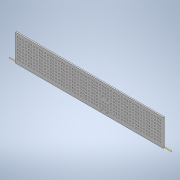
# Autodesk Inventor part: top_plate
Saved by Autodesk Inventor 2022 (Build 260153000, 153)
## iProperties
Created: 2021-07-14
Part Number: top_plate
Material: Generic
Document SubType Name: Modeling
Designer: gfellows
Density: 1 g/cm^3
Appearance: Default
Author: gfellows
Autodesk Inventor part; units mm, degrees
ref_plane "YZ Plane" through (0, 0, 0) normal (1, 0, 0) x (0, 1, 0)
ref_plane "XZ Plane" through (0, 0, 0) normal (0, 1, 0) x (-1, 0, 0)
ref_plane "XY Plane" through (0, 0, 0) normal (0, 0, 1) x (1, 0, 0)
ref_plane "Work Plane1" through (-371.7905, 0, 55) normal (0, 0, 1) x (1, 0, 0)
sketch "Sketch1" plane through (-371.7905, 0, 55) normal (0, 0, 1) x (1, 0, 0)
  line L0 (0, 0) -> (430.2, 0)
  line L1 (430.2, 0) -> (430.2, 78.35)
  line L2 (430.2, 78.35) -> (0, 78.35)
  line L3 (0, 78.35) -> (0, 0)
  circle A0 centre (265.5182, 6.225) radius 1.3525 projected
  line L4 (232.7522, 3.429) -> (232.7522, 41.021) projected
  line L5 (271.9952, 3.429) -> (232.7522, 3.429) projected
  line L6 (271.9952, 41.021) -> (271.9952, 3.429) projected
  line L7 (232.7522, 41.021) -> (271.9952, 41.021) projected
  circle A1 centre (265.5182, 6.225) radius 1.3525 projected
  circle A2 centre (249.5182, 6.225) radius 1.3525 projected
  circle A3 centre (265.5182, 38.225) radius 1.3525 projected
  circle A4 centre (249.5182, 38.225) radius 1.3525 projected
  circle A5 centre (5.8257, 12.35) radius 1.65
  line L8 (0, 75.175) -> (0, 78.35) projected
  line L9 (0, 0) -> (430.2, 0) projected
  circle A6 centre (5.8257, 20.35) radius 1.65
  circle A7 centre (5.8257, 28.35) radius 1.65
  circle A8 centre (5.8257, 36.35) radius 1.65
  circle A9 centre (5.8257, 44.35) radius 1.65
  circle A10 centre (5.8257, 52.35) radius 1.65
  circle A11 centre (5.8257, 60.35) radius 1.65
  circle A12 centre (5.8257, 68.35) radius 1.65
  circle A13 centre (13.8257, 12.35) radius 1.65
  circle A14 centre (13.8257, 20.35) radius 1.65
  circle A15 centre (13.8257, 28.35) radius 1.65
  circle A16 centre (13.8257, 36.35) radius 1.65
  circle A17 centre (13.8257, 44.35) radius 1.65
  circle A18 centre (13.8257, 52.35) radius 1.65
  circle A19 centre (13.8257, 60.35) radius 1.65
  circle A20 centre (13.8257, 68.35) radius 1.65
  circle A21 centre (21.8257, 12.35) radius 1.65
  circle A22 centre (21.8257, 20.35) radius 1.65
  circle A23 centre (21.8257, 28.35) radius 1.65
  circle A24 centre (21.8257, 36.35) radius 1.65
  circle A25 centre (21.8257, 44.35) radius 1.65
  circle A26 centre (21.8257, 52.35) radius 1.65
  circle A27 centre (21.8257, 60.35) radius 1.65
  circle A28 centre (21.8257, 68.35) radius 1.65
  circle A29 centre (29.8257, 12.35) radius 1.65
  circle A30 centre (29.8257, 20.35) radius 1.65
  circle A31 centre (29.8257, 28.35) radius 1.65
  circle A32 centre (29.8257, 36.35) radius 1.65
  circle A33 centre (29.8257, 44.35) radius 1.65
  circle A34 centre (29.8257, 52.35) radius 1.65
  circle A35 centre (29.8257, 60.35) radius 1.65
  circle A36 centre (29.8257, 68.35) radius 1.65
  circle A37 centre (37.8257, 12.35) radius 1.65
  circle A38 centre (37.8257, 20.35) radius 1.65
  circle A39 centre (37.8257, 28.35) radius 1.65
  circle A40 centre (37.8257, 36.35) radius 1.65
  circle A41 centre (37.8257, 44.35) radius 1.65
  circle A42 centre (37.8257, 52.35) radius 1.65
  circle A43 centre (37.8257, 60.35) radius 1.65
  circle A44 centre (37.8257, 68.35) radius 1.65
  circle A45 centre (45.8257, 12.35) radius 1.65
  circle A46 centre (45.8257, 20.35) radius 1.65
  circle A47 centre (45.8257, 28.35) radius 1.65
  circle A48 centre (45.8257, 36.35) radius 1.65
  circle A49 centre (45.8257, 44.35) radius 1.65
  circle A50 centre (45.8257, 52.35) radius 1.65
  circle A51 centre (45.8257, 60.35) radius 1.65
  circle A52 centre (45.8257, 68.35) radius 1.65
  circle A53 centre (53.8257, 12.35) radius 1.65
  circle A54 centre (53.8257, 20.35) radius 1.65
  circle A55 centre (53.8257, 28.35) radius 1.65
  circle A56 centre (53.8257, 36.35) radius 1.65
  circle A57 centre (53.8257, 44.35) radius 1.65
  circle A58 centre (53.8257, 52.35) radius 1.65
  circle A59 centre (53.8257, 60.35) radius 1.65
  circle A60 centre (53.8257, 68.35) radius 1.65
  circle A61 centre (61.8257, 12.35) radius 1.65
  circle A62 centre (61.8257, 20.35) radius 1.65
  circle A63 centre (61.8257, 28.35) radius 1.65
  circle A64 centre (61.8257, 36.35) radius 1.65
  circle A65 centre (61.8257, 44.35) radius 1.65
  circle A66 centre (61.8257, 52.35) radius 1.65
  circle A67 centre (61.8257, 60.35) radius 1.65
  circle A68 centre (61.8257, 68.35) radius 1.65
  circle A69 centre (69.8257, 12.35) radius 1.65
  circle A70 centre (69.8257, 20.35) radius 1.65
  circle A71 centre (69.8257, 28.35) radius 1.65
  circle A72 centre (69.8257, 36.35) radius 1.65
  circle A73 centre (69.8257, 44.35) radius 1.65
  circle A74 centre (69.8257, 52.35) radius 1.65
  circle A75 centre (69.8257, 60.35) radius 1.65
  circle A76 centre (69.8257, 68.35) radius 1.65
  circle A77 centre (77.8257, 12.35) radius 1.65
  circle A78 centre (77.8257, 20.35) radius 1.65
  circle A79 centre (77.8257, 28.35) radius 1.65
  circle A80 centre (77.8257, 36.35) radius 1.65
  circle A81 centre (77.8257, 44.35) radius 1.65
  circle A82 centre (77.8257, 52.35) radius 1.65
  circle A83 centre (77.8257, 60.35) radius 1.65
  circle A84 centre (77.8257, 68.35) radius 1.65
  circle A85 centre (85.8257, 12.35) radius 1.65
  circle A86 centre (85.8257, 20.35) radius 1.65
  circle A87 centre (85.8257, 28.35) radius 1.65
  circle A88 centre (85.8257, 36.35) radius 1.65
  circle A89 centre (85.8257, 44.35) radius 1.65
  circle A90 centre (85.8257, 52.35) radius 1.65
  circle A91 centre (85.8257, 60.35) radius 1.65
  circle A92 centre (85.8257, 68.35) radius 1.65
  circle A93 centre (93.8257, 12.35) radius 1.65
  circle A94 centre (93.8257, 20.35) radius 1.65
  circle A95 centre (93.8257, 28.35) radius 1.65
  circle A96 centre (93.8257, 36.35) radius 1.65
  circle A97 centre (93.8257, 44.35) radius 1.65
  circle A98 centre (93.8257, 52.35) radius 1.65
  circle A99 centre (93.8257, 60.35) radius 1.65
  circle A100 centre (93.8257, 68.35) radius 1.65
  circle A101 centre (101.8257, 12.35) radius 1.65
  circle A102 centre (101.8257, 20.35) radius 1.65
  circle A103 centre (101.8257, 28.35) radius 1.65
  circle A104 centre (101.8257, 36.35) radius 1.65
  circle A105 centre (101.8257, 44.35) radius 1.65
  circle A106 centre (101.8257, 52.35) radius 1.65
  circle A107 centre (101.8257, 60.35) radius 1.65
  circle A108 centre (101.8257, 68.35) radius 1.65
  circle A109 centre (109.8257, 12.35) radius 1.65
  circle A110 centre (109.8257, 20.35) radius 1.65
  circle A111 centre (109.8257, 28.35) radius 1.65
  circle A112 centre (109.8257, 36.35) radius 1.65
  circle A113 centre (109.8257, 44.35) radius 1.65
  circle A114 centre (109.8257, 52.35) radius 1.65
  circle A115 centre (109.8257, 60.35) radius 1.65
  circle A116 centre (109.8257, 68.35) radius 1.65
  circle A117 centre (117.8257, 12.35) radius 1.65
  circle A118 centre (117.8257, 20.35) radius 1.65
  circle A119 centre (117.8257, 28.35) radius 1.65
  circle A120 centre (117.8257, 36.35) radius 1.65
  circle A121 centre (117.8257, 44.35) radius 1.65
  circle A122 centre (117.8257, 52.35) radius 1.65
  circle A123 centre (117.8257, 60.35) radius 1.65
  circle A124 centre (117.8257, 68.35) radius 1.65
  circle A125 centre (125.8257, 12.35) radius 1.65
  circle A126 centre (125.8257, 20.35) radius 1.65
  circle A127 centre (125.8257, 28.35) radius 1.65
  circle A128 centre (125.8257, 36.35) radius 1.65
  circle A129 centre (125.8257, 44.35) radius 1.65
  circle A130 centre (125.8257, 52.35) radius 1.65
  circle A131 centre (125.8257, 60.35) radius 1.65
  circle A132 centre (125.8257, 68.35) radius 1.65
  circle A133 centre (133.8257, 12.35) radius 1.65
  circle A134 centre (133.8257, 20.35) radius 1.65
  circle A135 centre (133.8257, 28.35) radius 1.65
  circle A136 centre (133.8257, 36.35) radius 1.65
  circle A137 centre (133.8257, 44.35) radius 1.65
  circle A138 centre (133.8257, 52.35) radius 1.65
  circle A139 centre (133.8257, 60.35) radius 1.65
  circle A140 centre (133.8257, 68.35) radius 1.65
  circle A141 centre (141.8257, 12.35) radius 1.65
  circle A142 centre (141.8257, 20.35) radius 1.65
  circle A143 centre (141.8257, 28.35) radius 1.65
  circle A144 centre (141.8257, 36.35) radius 1.65
  circle A145 centre (141.8257, 44.35) radius 1.65
  circle A146 centre (141.8257, 52.35) radius 1.65
  circle A147 centre (141.8257, 60.35) radius 1.65
  circle A148 centre (141.8257, 68.35) radius 1.65
  circle A149 centre (149.8257, 12.35) radius 1.65
  circle A150 centre (149.8257, 20.35) radius 1.65
  circle A151 centre (149.8257, 28.35) radius 1.65
  circle A152 centre (149.8257, 36.35) radius 1.65
  circle A153 centre (149.8257, 44.35) radius 1.65
  circle A154 centre (149.8257, 52.35) radius 1.65
  circle A155 centre (149.8257, 60.35) radius 1.65
  circle A156 centre (149.8257, 68.35) radius 1.65
  circle A157 centre (157.8257, 12.35) radius 1.65
  circle A158 centre (157.8257, 20.35) radius 1.65
  circle A159 centre (157.8257, 28.35) radius 1.65
  circle A160 centre (157.8257, 36.35) radius 1.65
  circle A161 centre (157.8257, 44.35) radius 1.65
  circle A162 centre (157.8257, 52.35) radius 1.65
  circle A163 centre (157.8257, 60.35) radius 1.65
  circle A164 centre (157.8257, 68.35) radius 1.65
  circle A165 centre (165.8257, 12.35) radius 1.65
  circle A166 centre (165.8257, 20.35) radius 1.65
  circle A167 centre (165.8257, 28.35) radius 1.65
  circle A168 centre (165.8257, 36.35) radius 1.65
  circle A169 centre (165.8257, 44.35) radius 1.65
  circle A170 centre (165.8257, 52.35) radius 1.65
  circle A171 centre (165.8257, 60.35) radius 1.65
  circle A172 centre (165.8257, 68.35) radius 1.65
  circle A173 centre (173.8257, 12.35) radius 1.65
  circle A174 centre (173.8257, 20.35) radius 1.65
  circle A175 centre (173.8257, 28.35) radius 1.65
  circle A176 centre (173.8257, 36.35) radius 1.65
  circle A177 centre (173.8257, 44.35) radius 1.65
  circle A178 centre (173.8257, 52.35) radius 1.65
  circle A179 centre (173.8257, 60.35) radius 1.65
  circle A180 centre (173.8257, 68.35) radius 1.65
  circle A181 centre (181.8257, 12.35) radius 1.65
  circle A182 centre (181.8257, 20.35) radius 1.65
  circle A183 centre (181.8257, 28.35) radius 1.65
  circle A184 centre (181.8257, 36.35) radius 1.65
  circle A185 centre (181.8257, 44.35) radius 1.65
  circle A186 centre (181.8257, 52.35) radius 1.65
  circle A187 centre (181.8257, 60.35) radius 1.65
  circle A188 centre (181.8257, 68.35) radius 1.65
  circle A189 centre (189.8257, 12.35) radius 1.65
  circle A190 centre (189.8257, 20.35) radius 1.65
  circle A191 centre (189.8257, 28.35) radius 1.65
  circle A192 centre (189.8257, 36.35) radius 1.65
  circle A193 centre (189.8257, 44.35) radius 1.65
  circle A194 centre (189.8257, 52.35) radius 1.65
  circle A195 centre (189.8257, 60.35) radius 1.65
  circle A196 centre (189.8257, 68.35) radius 1.65
  circle A197 centre (197.8257, 12.35) radius 1.65
  circle A198 centre (197.8257, 20.35) radius 1.65
  circle A199 centre (197.8257, 28.35) radius 1.65
  circle A200 centre (197.8257, 36.35) radius 1.65
  circle A201 centre (197.8257, 44.35) radius 1.65
  circle A202 centre (197.8257, 52.35) radius 1.65
  circle A203 centre (197.8257, 60.35) radius 1.65
  circle A204 centre (197.8257, 68.35) radius 1.65
  circle A205 centre (205.8257, 12.35) radius 1.65
  circle A206 centre (205.8257, 20.35) radius 1.65
  circle A207 centre (205.8257, 28.35) radius 1.65
  circle A208 centre (205.8257, 36.35) radius 1.65
  circle A209 centre (205.8257, 44.35) radius 1.65
  circle A210 centre (205.8257, 52.35) radius 1.65
  circle A211 centre (205.8257, 60.35) radius 1.65
  circle A212 centre (205.8257, 68.35) radius 1.65
  circle A213 centre (213.8257, 12.35) radius 1.65
  circle A214 centre (213.8257, 20.35) radius 1.65
  circle A215 centre (213.8257, 28.35) radius 1.65
  circle A216 centre (213.8257, 36.35) radius 1.65
  circle A217 centre (213.8257, 44.35) radius 1.65
  circle A218 centre (213.8257, 52.35) radius 1.65
  circle A219 centre (213.8257, 60.35) radius 1.65
  circle A220 centre (213.8257, 68.35) radius 1.65
  circle A221 centre (221.8257, 12.35) radius 1.65
  circle A222 centre (221.8257, 20.35) radius 1.65
  circle A223 centre (221.8257, 28.35) radius 1.65
  circle A224 centre (221.8257, 36.35) radius 1.65
  circle A225 centre (221.8257, 44.35) radius 1.65
  circle A226 centre (221.8257, 52.35) radius 1.65
  circle A227 centre (221.8257, 60.35) radius 1.65
  circle A228 centre (221.8257, 68.35) radius 1.65
  circle A229 centre (229.8257, 12.35) radius 1.65
  circle A230 centre (229.8257, 20.35) radius 1.65
  circle A231 centre (229.8257, 28.35) radius 1.65
  circle A232 centre (229.8257, 36.35) radius 1.65
  circle A233 centre (229.8257, 44.35) radius 1.65
  circle A234 centre (229.8257, 52.35) radius 1.65
  circle A235 centre (229.8257, 60.35) radius 1.65
  circle A236 centre (229.8257, 68.35) radius 1.65
  circle A237 centre (237.8257, 12.35) radius 1.65
  circle A238 centre (237.8257, 20.35) radius 1.65
  circle A239 centre (237.8257, 28.35) radius 1.65
  circle A240 centre (237.8257, 36.35) radius 1.65
  circle A241 centre (237.8257, 44.35) radius 1.65
  circle A242 centre (237.8257, 52.35) radius 1.65
  circle A243 centre (237.8257, 60.35) radius 1.65
  circle A244 centre (237.8257, 68.35) radius 1.65
  circle A245 centre (245.8257, 12.35) radius 1.65
  circle A246 centre (245.8257, 20.35) radius 1.65
  circle A247 centre (245.8257, 28.35) radius 1.65
  circle A248 centre (245.8257, 36.35) radius 1.65
  circle A249 centre (245.8257, 44.35) radius 1.65
  circle A250 centre (245.8257, 52.35) radius 1.65
  circle A251 centre (245.8257, 60.35) radius 1.65
  circle A252 centre (245.8257, 68.35) radius 1.65
  circle A253 centre (253.8257, 12.35) radius 1.65
  circle A254 centre (253.8257, 20.35) radius 1.65
  circle A255 centre (253.8257, 28.35) radius 1.65
  circle A256 centre (253.8257, 36.35) radius 1.65
  circle A257 centre (253.8257, 44.35) radius 1.65
  circle A258 centre (253.8257, 52.35) radius 1.65
  circle A259 centre (253.8257, 60.35) radius 1.65
  circle A260 centre (253.8257, 68.35) radius 1.65
  circle A261 centre (261.8257, 12.35) radius 1.65
  circle A262 centre (261.8257, 20.35) radius 1.65
  circle A263 centre (261.8257, 28.35) radius 1.65
  circle A264 centre (261.8257, 36.35) radius 1.65
  circle A265 centre (261.8257, 44.35) radius 1.65
  circle A266 centre (261.8257, 52.35) radius 1.65
  circle A267 centre (261.8257, 60.35) radius 1.65
  circle A268 centre (261.8257, 68.35) radius 1.65
  circle A269 centre (269.8257, 12.35) radius 1.65
  circle A270 centre (269.8257, 20.35) radius 1.65
  circle A271 centre (269.8257, 28.35) radius 1.65
  circle A272 centre (269.8257, 36.35) radius 1.65
  circle A273 centre (269.8257, 44.35) radius 1.65
  circle A274 centre (269.8257, 52.35) radius 1.65
  circle A275 centre (269.8257, 60.35) radius 1.65
  circle A276 centre (269.8257, 68.35) radius 1.65
  circle A277 centre (277.8257, 12.35) radius 1.65
  circle A278 centre (277.8257, 20.35) radius 1.65
  circle A279 centre (277.8257, 28.35) radius 1.65
  circle A280 centre (277.8257, 36.35) radius 1.65
  circle A281 centre (277.8257, 44.35) radius 1.65
  circle A282 centre (277.8257, 52.35) radius 1.65
  circle A283 centre (277.8257, 60.35) radius 1.65
  circle A284 centre (277.8257, 68.35) radius 1.65
  circle A285 centre (285.8257, 12.35) radius 1.65
  circle A286 centre (285.8257, 20.35) radius 1.65
  circle A287 centre (285.8257, 28.35) radius 1.65
  circle A288 centre (285.8257, 36.35) radius 1.65
  circle A289 centre (285.8257, 44.35) radius 1.65
  circle A290 centre (285.8257, 52.35) radius 1.65
  circle A291 centre (285.8257, 60.35) radius 1.65
  circle A292 centre (285.8257, 68.35) radius 1.65
  circle A293 centre (293.8257, 12.35) radius 1.65
  circle A294 centre (293.8257, 20.35) radius 1.65
  circle A295 centre (293.8257, 28.35) radius 1.65
  circle A296 centre (293.8257, 36.35) radius 1.65
  circle A297 centre (293.8257, 44.35) radius 1.65
  circle A298 centre (293.8257, 52.35) radius 1.65
  circle A299 centre (293.8257, 60.35) radius 1.65
  circle A300 centre (293.8257, 68.35) radius 1.65
  circle A301 centre (301.8257, 12.35) radius 1.65
  circle A302 centre (301.8257, 20.35) radius 1.65
  circle A303 centre (301.8257, 28.35) radius 1.65
  circle A304 centre (301.8257, 36.35) radius 1.65
  circle A305 centre (301.8257, 44.35) radius 1.65
  circle A306 centre (301.8257, 52.35) radius 1.65
  circle A307 centre (301.8257, 60.35) radius 1.65
  circle A308 centre (301.8257, 68.35) radius 1.65
  circle A309 centre (309.8257, 12.35) radius 1.65
  circle A310 centre (309.8257, 20.35) radius 1.65
  circle A311 centre (309.8257, 28.35) radius 1.65
  circle A312 centre (309.8257, 36.35) radius 1.65
  circle A313 centre (309.8257, 44.35) radius 1.65
  circle A314 centre (309.8257, 52.35) radius 1.65
  circle A315 centre (309.8257, 60.35) radius 1.65
  circle A316 centre (309.8257, 68.35) radius 1.65
  circle A317 centre (317.8257, 12.35) radius 1.65
  circle A318 centre (317.8257, 20.35) radius 1.65
  circle A319 centre (317.8257, 28.35) radius 1.65
  circle A320 centre (317.8257, 36.35) radius 1.65
  circle A321 centre (317.8257, 44.35) radius 1.65
  circle A322 centre (317.8257, 52.35) radius 1.65
  circle A323 centre (317.8257, 60.35) radius 1.65
  circle A324 centre (317.8257, 68.35) radius 1.65
  circle A325 centre (325.8257, 12.35) radius 1.65
  circle A326 centre (325.8257, 20.35) radius 1.65
  circle A327 centre (325.8257, 28.35) radius 1.65
  circle A328 centre (325.8257, 36.35) radius 1.65
  circle A329 centre (325.8257, 44.35) radius 1.65
  circle A330 centre (325.8257, 52.35) radius 1.65
  circle A331 centre (325.8257, 60.35) radius 1.65
  circle A332 centre (325.8257, 68.35) radius 1.65
  circle A333 centre (333.8257, 12.35) radius 1.65
  circle A334 centre (333.8257, 20.35) radius 1.65
  circle A335 centre (333.8257, 28.35) radius 1.65
  circle A336 centre (333.8257, 36.35) radius 1.65
  circle A337 centre (333.8257, 44.35) radius 1.65
  circle A338 centre (333.8257, 52.35) radius 1.65
  circle A339 centre (333.8257, 60.35) radius 1.65
  circle A340 centre (333.8257, 68.35) radius 1.65
  circle A341 centre (341.8257, 12.35) radius 1.65
  circle A342 centre (341.8257, 20.35) radius 1.65
  circle A343 centre (341.8257, 28.35) radius 1.65
  circle A344 centre (341.8257, 36.35) radius 1.65
  circle A345 centre (341.8257, 44.35) radius 1.65
  circle A346 centre (341.8257, 52.35) radius 1.65
  circle A347 centre (341.8257, 60.35) radius 1.65
  circle A348 centre (341.8257, 68.35) radius 1.65
  circle A349 centre (349.8257, 12.35) radius 1.65
  circle A350 centre (349.8257, 20.35) radius 1.65
  circle A351 centre (349.8257, 28.35) radius 1.65
  circle A352 centre (349.8257, 36.35) radius 1.65
  circle A353 centre (349.8257, 44.35) radius 1.65
  circle A354 centre (349.8257, 52.35) radius 1.65
  circle A355 centre (349.8257, 60.35) radius 1.65
  circle A356 centre (349.8257, 68.35) radius 1.65
  circle A357 centre (357.8257, 12.35) radius 1.65
  circle A358 centre (357.8257, 20.35) radius 1.65
  circle A359 centre (357.8257, 28.35) radius 1.65
  circle A360 centre (357.8257, 36.35) radius 1.65
  circle A361 centre (357.8257, 44.35) radius 1.65
  circle A362 centre (357.8257, 52.35) radius 1.65
  circle A363 centre (357.8257, 60.35) radius 1.65
  circle A364 centre (357.8257, 68.35) radius 1.65
  circle A365 centre (365.8257, 12.35) radius 1.65
  circle A366 centre (365.8257, 20.35) radius 1.65
  circle A367 centre (365.8257, 28.35) radius 1.65
  circle A368 centre (365.8257, 36.35) radius 1.65
  circle A369 centre (365.8257, 44.35) radius 1.65
  circle A370 centre (365.8257, 52.35) radius 1.65
  circle A371 centre (365.8257, 60.35) radius 1.65
  circle A372 centre (365.8257, 68.35) radius 1.65
  circle A373 centre (373.8257, 12.35) radius 1.65
  circle A374 centre (373.8257, 20.35) radius 1.65
  circle A375 centre (373.8257, 28.35) radius 1.65
  circle A376 centre (373.8257, 36.35) radius 1.65
  circle A377 centre (373.8257, 44.35) radius 1.65
  circle A378 centre (373.8257, 52.35) radius 1.65
  circle A379 centre (373.8257, 60.35) radius 1.65
  circle A380 centre (373.8257, 68.35) radius 1.65
  circle A381 centre (381.8257, 12.35) radius 1.65
  circle A382 centre (381.8257, 20.35) radius 1.65
  circle A383 centre (381.8257, 28.35) radius 1.65
  circle A384 centre (381.8257, 36.35) radius 1.65
  circle A385 centre (381.8257, 44.35) radius 1.65
  circle A386 centre (381.8257, 52.35) radius 1.65
  circle A387 centre (381.8257, 60.35) radius 1.65
  circle A388 centre (381.8257, 68.35) radius 1.65
  circle A389 centre (389.8257, 12.35) radius 1.65
  circle A390 centre (389.8257, 20.35) radius 1.65
  circle A391 centre (389.8257, 28.35) radius 1.65
  circle A392 centre (389.8257, 36.35) radius 1.65
  circle A393 centre (389.8257, 44.35) radius 1.65
  circle A394 centre (389.8257, 52.35) radius 1.65
  circle A395 centre (389.8257, 60.35) radius 1.65
  circle A396 centre (389.8257, 68.35) radius 1.65
  circle A397 centre (397.8257, 12.35) radius 1.65
  circle A398 centre (397.8257, 20.35) radius 1.65
  circle A399 centre (397.8257, 28.35) radius 1.65
  circle A400 centre (397.8257, 36.35) radius 1.65
  circle A401 centre (397.8257, 44.35) radius 1.65
  circle A402 centre (397.8257, 52.35) radius 1.65
  circle A403 centre (397.8257, 60.35) radius 1.65
  circle A404 centre (397.8257, 68.35) radius 1.65
  circle A405 centre (405.8257, 12.35) radius 1.65
  circle A406 centre (405.8257, 20.35) radius 1.65
  circle A407 centre (405.8257, 28.35) radius 1.65
  circle A408 centre (405.8257, 36.35) radius 1.65
  circle A409 centre (405.8257, 44.35) radius 1.65
  circle A410 centre (405.8257, 52.35) radius 1.65
  circle A411 centre (405.8257, 60.35) radius 1.65
  circle A412 centre (405.8257, 68.35) radius 1.65
  circle A413 centre (413.8257, 12.35) radius 1.65
  circle A414 centre (413.8257, 20.35) radius 1.65
  circle A415 centre (413.8257, 28.35) radius 1.65
  circle A416 centre (413.8257, 36.35) radius 1.65
  circle A417 centre (413.8257, 44.35) radius 1.65
  circle A418 centre (413.8257, 52.35) radius 1.65
  circle A419 centre (413.8257, 60.35) radius 1.65
  circle A420 centre (413.8257, 68.35) radius 1.65
  circle A421 centre (421.8257, 12.35) radius 1.65
  circle A422 centre (421.8257, 20.35) radius 1.65
  circle A423 centre (421.8257, 28.35) radius 1.65
  circle A424 centre (421.8257, 36.35) radius 1.65
  circle A425 centre (421.8257, 44.35) radius 1.65
  circle A426 centre (421.8257, 52.35) radius 1.65
  circle A427 centre (421.8257, 60.35) radius 1.65
  circle A428 centre (421.8257, 68.35) radius 1.65
  line L10 (0, 78.35) -> (430.2, 78.35) projected
  line L11 (120.0709, 342.35) -> (109.0209, 342.35) projected
  line L12 (120.0709, 342.35) -> (120.0709, 78.35)
  line L13 (120.0709, 210.35) -> (0, 210.35)
  line L14 (0, 75.175) -> (0, 63.175) projected
  line L15 (280, 63.175) -> (0, 63.175) projected
  line L16 (280, 75.175) -> (280, 63.175) projected
  line L17 (280, 75.175) -> (0, 75.175) projected
  circle A429 centre (4, 67.175) radius 2 projected
  circle A430 centre (12, 67.175) radius 2 projected
  circle A431 centre (20, 67.175) radius 2 projected
  circle A432 centre (28, 67.175) radius 2 projected
  circle A433 centre (36, 67.175) radius 2 projected
  circle A434 centre (44, 67.175) radius 2 projected
  circle A435 centre (52, 67.175) radius 2 projected
  circle A436 centre (60, 67.175) radius 2 projected
  circle A437 centre (68, 67.175) radius 2 projected
  circle A438 centre (76, 67.175) radius 2 projected
  circle A439 centre (84, 67.175) radius 2 projected
  circle A440 centre (92, 67.175) radius 2 projected
  circle A441 centre (100, 67.175) radius 2 projected
  circle A442 centre (108, 67.175) radius 2 projected
  circle A443 centre (116, 67.175) radius 2 projected
  circle A444 centre (124, 67.175) radius 2 projected
  circle A445 centre (132, 67.175) radius 2 projected
  circle A446 centre (140, 67.175) radius 2 projected
  circle A447 centre (148, 67.175) radius 2 projected
  circle A448 centre (156, 67.175) radius 2 projected
  circle A449 centre (164, 67.175) radius 2 projected
  circle A450 centre (172, 67.175) radius 2 projected
  circle A451 centre (180, 67.175) radius 2 projected
  circle A452 centre (188, 67.175) radius 2 projected
  circle A453 centre (196, 67.175) radius 2 projected
  circle A454 centre (204, 67.175) radius 2 projected
  circle A455 centre (212, 67.175) radius 2 projected
  circle A456 centre (220, 67.175) radius 2 projected
  circle A457 centre (228, 67.175) radius 2 projected
  circle A458 centre (236, 67.175) radius 2 projected
  circle A459 centre (244, 67.175) radius 2 projected
  circle A460 centre (252, 67.175) radius 2 projected
  circle A461 centre (260, 67.175) radius 2 projected
  circle A462 centre (268, 67.175) radius 2 projected
  circle A463 centre (276, 67.175) radius 2 projected
  line L18 (342.2, 75.175) -> (342.2, 63.175) projected
  line L19 (430.2, 63.175) -> (342.2, 63.175) projected
  line L20 (430.2, 75.175) -> (430.2, 63.175) projected
  line L21 (430.2, 75.175) -> (342.2, 75.175) projected
  circle A464 centre (346.2, 67.175) radius 2 projected
  circle A465 centre (354.2, 67.175) radius 2 projected
  circle A466 centre (362.2, 67.175) radius 2 projected
  circle A467 centre (370.2, 67.175) radius 2 projected
  circle A468 centre (378.2, 67.175) radius 2 projected
  circle A469 centre (386.2, 67.175) radius 2 projected
  circle A470 centre (394.2, 67.175) radius 2 projected
  circle A471 centre (402.2, 67.175) radius 2 projected
  circle A472 centre (410.2, 67.175) radius 2 projected
  circle A473 centre (418.2, 67.175) radius 2 projected
  circle A474 centre (426.2, 67.175) radius 2 projected
  line L22 (342.2, 3.175) -> (342.2, 15.175) projected
  line L23 (430.2, 3.175) -> (342.2, 3.175) projected
  line L24 (430.2, 3.175) -> (430.2, 15.175) projected
  line L25 (430.2, 15.175) -> (342.2, 15.175) projected
  circle A475 centre (362.2, 11.175) radius 2 projected
  circle A476 centre (370.2, 11.175) radius 2 projected
  circle A477 centre (378.2, 11.175) radius 2 projected
  circle A478 centre (386.2, 11.175) radius 2 projected
  circle A479 centre (394.2, 11.175) radius 2 projected
  circle A480 centre (402.2, 11.175) radius 2 projected
  circle A481 centre (410.2, 11.175) radius 2 projected
  circle A482 centre (418.2, 11.175) radius 2 projected
  circle A483 centre (426.2, 11.175) radius 2 projected
  circle A484 centre (354.2, 11.175) radius 2 projected
  circle A485 centre (346.2, 11.175) radius 2 projected
  line L26 (0, 3.175) -> (0, 15.175) projected
  line L27 (88, 3.175) -> (0, 3.175) projected
  line L28 (88, 3.175) -> (88, 15.175) projected
  line L29 (88, 15.175) -> (0, 15.175) projected
  circle A486 centre (20, 11.175) radius 2 projected
  circle A487 centre (28, 11.175) radius 2 projected
  circle A488 centre (36, 11.175) radius 2 projected
  circle A489 centre (44, 11.175) radius 2 projected
  circle A490 centre (52, 11.175) radius 2 projected
  circle A491 centre (60, 11.175) radius 2 projected
  circle A492 centre (68, 11.175) radius 2 projected
  circle A493 centre (76, 11.175) radius 2 projected
  circle A494 centre (84, 11.175) radius 2 projected
  circle A495 centre (12, 11.175) radius 2 projected
  circle A496 centre (4, 11.175) radius 2 projected
  point P0 (371.7905, 0)
  point P1 (118.0382, 342.35)
  dimension "d7" = 3.3
  dimension "d10" = 8
  dimension "d13" = 8
  dimension "d16" = 142
  constraints: 424 centre point, 12 end point, 3 horizontal, 2 parallel, 2 perpendicular, 1 midpoint, 1 point on line, 1 vertical, 849 other
  measures "d7" diameter of A5
  measures "d10" distance of A5.centre A6.centre
  measures "d13" distance of A5.centre A13.centre
  measures "d16" distance from line of L13 A12.centre
extrude "Extrusion1" add sketch "Sketch1" along normal blind 3.175 contours L3 L27 L28 L29 L15 L16 L17 L2 L1 L21 L18 A348 L19 L25 L22 A341 L23 L0 | L3 L29 L28 L27 | L23 L22 A341 L25 L1 | L3 L17 L16 L15 | L19 L18 A348 L21 L1 | L22 A341 | A341 L22 | L18 A348 | A348 L18 | L4 L7 L6 L5 | A5 A496 | A12 A429 | A13 A495 | A20 A430 | A21 A486 | A28 A431 | A29 A487 | A36 A432 | A37 A488 | A44 A433 | A45 A489 | A52 A434 | A53 A490 | A60 A435 | A61 A491 | A68 A436 | A69 A492 | A76 A437 | A77 A493 | A84 A438 | A85 A494 | A92 A439 | A100 A440 | A108 A441 | A116 A442 | A124 A443 | A132 A444 | A140 A445 | A148 A446 | A156 A447 | A164 A448 | A172 A449 | A180 A450 | A188 A451 | A196 A452 | A204 A453 | A212 A454 | A220 A455 | A228 A456 | A236 A457 | A244 A458 | A248 | A252 A459 | A256 | A260 A460 | A264 | A268 A461 | A272 | A276 A462 | A284 A463 | A349 | A356 | A357 | A364 | A365 | A372 | A373 | A380 | A381 | A388 | A389 | A396 | A397 | A404 | A405 | A412 | A413 | A420 | A421 | A428 picked at (6.2074, 12.5418) picked at (6.2074, 68.5418) picked at (14.2074, 12.5418) picked at (14.2074, 68.5418) picked at (22.2074, 12.5418) picked at (22.2074, 68.5418) picked at (30.2074, 12.5418) picked at (30.2074, 68.5418) picked at (38.2074, 12.5418) picked at (38.2074, 68.5418) picked at (46.2074, 12.5418) picked at (46.2074, 68.5418) picked at (54.2074, 12.5418) picked at (54.2074, 68.5418) picked at (62.2074, 12.5418) picked at (62.2074, 68.5418) picked at (70.2074, 12.5418) picked at (70.2074, 68.5418) picked at (78.2074, 12.5418) picked at (78.2074, 68.5418) picked at (86.2074, 12.5418) picked at (86.2074, 68.5418) picked at (91.0013, 66.6098) picked at (99.0013, 66.6098) picked at (107.0013, 66.6098) picked at (115.0013, 66.6098) picked at (123.0013, 66.6098) picked at (131.0719, 66.5001) picked at (139.0719, 66.5001) picked at (147.0719, 66.5001) picked at (155.0719, 66.5001) picked at (163.0719, 66.5001) picked at (171.0719, 66.5001) picked at (179.0719, 66.5001) picked at (190.2074, 68.5418) picked at (198.2074, 68.5418) picked at (206.2074, 68.5418) picked at (214.2074, 68.5418) picked at (222.2074, 68.5418) picked at (230.2074, 68.5418) picked at (238.2074, 68.5418) picked at (246.2074, 68.5418) picked at (254.2074, 68.5418) picked at (262.2074, 68.5418) picked at (270.2074, 68.5418) picked at (275.0013, 66.6098)
body "Solid1"
